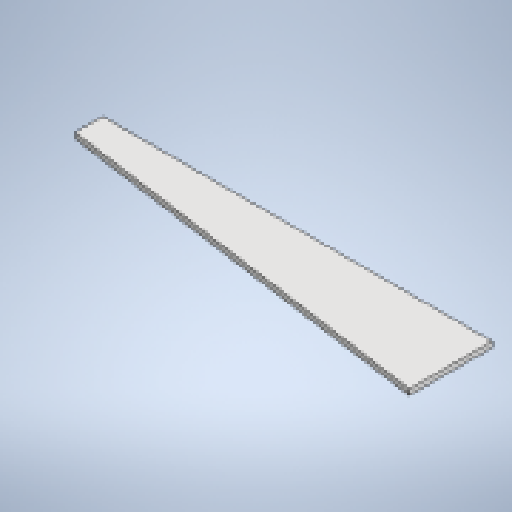
# Autodesk Inventor part: TRM 030 star conrtforce plate
Saved by Autodesk Inventor 2025 (Build 290162010, 162A)
## iProperties
Created: 2024-08-07
Part Number: TRM 030 star conrtforce plate
Material: AISI 304
Document SubType Name: Sheet Metal
Designer: admin
Stock Number: ТРМ 015 левый борт основное
Density: 8.02768 g/cm^3
Flat Pattern Width: 14.1 cm
Flat Pattern Length: 3 cm
Flat Pattern Area: 42.3 cm^2
Sheet Metal Rule: AISI304 2mm Die16
Sheet Metal Width: 141,000 mm
Sheet Metal Length: 30,000 mm
Sheet Metal Area: 4230,000 mm^2
Appearance: Default
Author: pokla
Autodesk Inventor part; units mm, degrees
ref_plane "YZ Plane" through (0, 0, 0) normal (1, 0, 0) x (0, 1, 0)
ref_plane "XZ Plane" through (0, 0, 0) normal (0, 1, 0) x (-1, 0, 0)
ref_plane "XY Plane" through (0, 0, 0) normal (0, 0, 1) x (1, 0, 0)
sketch "Sketch1" plane through (0, 0, 0) normal (0, 0, 1) x (1, 0, 0)
  line L0 (141, 0) -> (141, -30)
  line L1 (141, 0) -> (0, 0)
  line L2 (0, 0) -> (0, -10)
  line L3 (0, -10) -> (141, -30)
  dimension "d42" = 30
  dimension "d43" = 10
  dimension "d44" = 141
  measures "d42" distance of L0.start L0.end
  measures "d43" distance of L1.end L2.end
  measures "d44" distance of L0.start L1.end
extrude "Plate1" add sketch "Sketch1" along normal blind 2
sketch "Sketch2" plane through (0, 0, 0) normal (0, 0, -1) x (-1, 0, 0)
  line L0 (-139.4183, -5.1276) -> (60.5817, -5.1276) construction
  line L1 (60.5817, -5.1276) -> (60.5817, -25.1276) construction
  line L2 (60.5817, -25.1276) -> (-139.4183, -25.1276) construction
  line L3 (-139.4183, -25.1276) -> (-139.4183, -5.1276) construction
  point P0 (0, 0)
  point P1 (-251, -525)
  dimension "d6" = 200
  dimension "d9" = 20
  constraints: 2 other
  measures "d6" distance of L0.start L0.end
  measures "d9" distance of L0.end L1.end
mark "Mark1"
equation "\"d2\" = Thickness"
equation "\"BendReliefWidth\" = Thickness"
equation "\"BendReliefDepth\" = 0.5 * Thickness"
equation "\"CornerReliefSize\" = 4 * Thickness"
equation "\"MinimumRemnant\" = 2 * Thickness"
equation "\"TransitionRadius\" = BendRadius"
equation "\"JacobiRadiusSize\" = BendRadius"
equation "\"GapSize\" = Thickness"
equation "\"Thickness\" = 2"
equation "\"BendRadius\" = 2.75"
body "Solid1"
